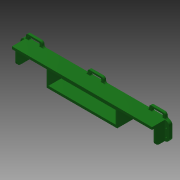
# Autodesk Inventor part: arm1
Saved by Autodesk Inventor 2013 (Build 170138000, 138)
## iProperties
Created: 2014-06-28
Part Number: arm1
Material: Generic
Document SubType Name: Modeling
Designer: Masta
Density: 1 g/cm^3
Author: Masta
Autodesk Inventor part; units mm, degrees
ref_plane "YZ Plane" through (0, 0, 0) normal (1, 0, 0) x (0, 1, 0)
ref_plane "XZ Plane" through (0, 0, 0) normal (0, 1, 0) x (-1, 0, 0)
ref_plane "XY Plane" through (0, 0, 0) normal (0, 0, 1) x (1, 0, 0)
sketch "Sketch2" plane through (0, 0, 0) normal (0, 0, 1) x (1, 0, 0)
  line L0 (0, 0) -> (186, 0)
  line L1 (186, 0) -> (186, 20)
  line L2 (186, 20) -> (0, 20)
  line L3 (0, 20) -> (0, 0)
  line L4 (178.5, 20) -> (178.5, 0)
  line L5 (7.5, 20) -> (7.5, 0)
  line L6 (49, 20) -> (49, 0)
  line L7 (137, 20) -> (137, 0)
  line L8 (0, 16) -> (7.5, 16)
  line L9 (49, 16) -> (137, 16)
  line L10 (178.5, 16) -> (186, 16)
  line L11 (135, 16) -> (135, 0)
  line L12 (180.5, 16) -> (180.5, 0)
  line L13 (51, 16) -> (51, 0)
  line L14 (5.5, 16) -> (5.5, 0)
  line L15 (178.5, 4) -> (180.5, 4)
  line L16 (5.5, 4) -> (7.5, 4)
  dimension "d17" = 186
  dimension "d18" = 20
  dimension "d19" = 7.5
  dimension "d20" = 7.5
  dimension "d21" = 41.5
  dimension "d22" = 41.5
  dimension "d23" = 4
  dimension "d26" = 2
  dimension "d27" = 2
  dimension "d28" = 2
  dimension "d29" = 2
  dimension "d46" = 12
  constraints: 32 end point, 18 point on line, 9 vertical, 4 collinear, 4 perpendicular, 1 horizontal, 1 parallel, 11 other
  measures "d17" distance of L2.end L1.end
  measures "d18" distance of L1.end L1.start
  measures "d19" distance between parallel lines of L3 L5
  measures "d20" distance between parallel lines of L1 L4
  measures "d21" distance between parallel lines of L6 L5
  measures "d22" distance between parallel lines of L4 L7
  measures "d23" distance between parallel lines of L2 L10
  measures "d26" distance between parallel lines of L5 L14
  measures "d27" distance between parallel lines of L6 L13
  measures "d28" distance between parallel lines of L7 L11
  measures "d29" distance between parallel lines of L4 L12
  measures "d46" distance between parallel lines of L8 L16
extrude "Extrusion1" add sketch "Sketch2" along normal blind 3 contours L14 L16 L5 L0 | L3 L2 L5 L8 | L5 L2 L6 L0 | L14 L8 L5 L16 | L6 L9 L13 L0 | L13 L9 L11 L0 | L6 L2 L7 L9 | L11 L9 L7 L0 | L2 L4 L0 L7 | L2 L1 L10 L4 | L4 L15 L12 L0 | L10 L12 L15 L4
extrude "Extrusion2" add sketch "Sketch2" against normal blind 20 contours L3 L2 L5 L8 | L14 L8 L5 L16 | L6 L9 L13 L0 | L6 L2 L7 L9 | L11 L9 L7 L0 | L2 L1 L10 L4 | L10 L12 L15 L4
sketch "Sketch3" plane through (0, 20, 3) normal (0, 1, 0) x (1, 0, 0)
  line L0 (7.5, 23) -> (49, 3) construction
  line L1 (137, 23) -> (178.5, 3) construction
  line L2 (52.5, 18) -> (4, 18) construction
  line L3 (4, 18) -> (4, 8) construction
  line L4 (4, 8) -> (52.5, 8) construction
  line L5 (52.5, 8) -> (52.5, 18) construction
  line L6 (52.5, 18) -> (4, 8) construction
  line L7 (4, 18) -> (52.5, 8) construction
  line L8 (133.5, 8) -> (182, 8) construction
  line L9 (182, 8) -> (182, 18) construction
  line L10 (182, 18) -> (133.5, 18) construction
  line L11 (133.5, 18) -> (133.5, 8) construction
  line L12 (133.5, 8) -> (182, 18) construction
  line L13 (182, 8) -> (133.5, 18) construction
  point P0 (0, 3)
  point P1 (28.25, 13)
  point P2 (157.75, 13)
  dimension "d32" = 48.5
  dimension "d33" = 10
  dimension "d34" = 48.5
  dimension "d35" = 10
  constraints: 28 end point, 8 coincident, 6 midpoint, 5 parallel, 2 horizontal, 2 perpendicular
  measures "d32" distance of L4.end L3.end
  measures "d33" distance of L3.end L2.end
  measures "d34" distance of L10.end L9.end
  measures "d35" distance of L9.end L8.end
hole "Hole1" at (4, 20, -5) at (4, 20, -15) at (52.5, 20, -15) at (52.5, 20, -5) at (133.5, 20, -15) at (133.5, 20, -5) at (182, 20, -15) at (182, 20, -5) direction (0, -1, 0) diameter 2 depth 8 tip angle 118
sketch "Sketch4" plane through (51, 16, -20) normal (0, -1, 0) x (1, 0, 0)
  line L0 (0, 20) -> (0, 0) projected
  line L1 (84, 0) -> (0, 0) projected
  line L2 (84, 20) -> (84, 0) projected
  line L3 (84, 3) -> (0, 3)
  point P0 (-51, 20)
  dimension "d43" = 3
  constraints: 2 end point, 2 point on line, 1 perpendicular
  measures "d43" distance between parallel lines of L1 L3
extrude "Extrusion3" add sketch "Sketch4" along normal up to surface (16 mm away)
fillet "Fillet1" radius 5 6 edges at (6.5, 4, -20) (179.5, 4, -20) (186, 18, -20) (0, 18, -20) (0, 18, 3) (186, 18, 3)
sketch "Sketch5" plane through (137, 20, 0) normal (0, 1, 0) x (1, 0, 0)
  line L0 (-137, 2) -> (-137, 15) projected
  line L1 (44, -3) -> (-132, -3) projected
  line L2 (-131, -3) -> (-111, -3)
  line L3 (-111, -3) -> (-111, -9)
  line L4 (-111, -9) -> (-131, -9)
  line L5 (-131, -9) -> (-131, -3)
  line L6 (-128, -3) -> (-114, -3)
  line L7 (-114, -3) -> (-114, -7)
  line L8 (-114, -7) -> (-128, -7)
  line L9 (-128, -7) -> (-128, -3)
  point P0 (-137, 0)
  dimension "d48" = 20
  dimension "d49" = 6
  dimension "d50" = 14
  dimension "d51" = 4
  dimension "d52" = 3
  dimension "d53" = 6
  constraints: 16 end point, 4 parallel, 2 horizontal, 2 perpendicular, 2 point on line
  measures "d48" distance of L3.end L4.end
  measures "d49" distance of L2.end L3.end
  measures "d50" distance of L7.end L8.end
  measures "d51" distance of L6.end L7.end
  measures "d52" distance between parallel lines of L5 L9
  measures "d53" distance between parallel lines of L0 L5
extrude "Extrusion4" add sketch "Sketch5" against normal blind 3 contours L3 L4 L5 L1 L9 L8 L7
fillet "Fillet2" radius 2.5 4 edges at (6, 18.5, 9) (6, 18.5, 3) (26, 18.5, 3) (26, 18.5, 9)
fillet "Fillet3" radius 1 4 edges at (23, 18.5, 7) (9, 18.5, 7) (9, 18.5, 3) (23, 18.5, 3)
pattern_linear "Rectangular Pattern1" count 3 spacing 77 along (1, 0, 0) of "Extrusion4", "Fillet2", "Fillet3"
body "Solid1"
